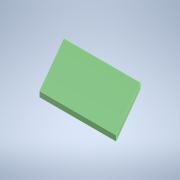
# Autodesk Inventor part: FactionSpecial_Council_Homel
Saved by Autodesk Inventor 2021 (Build 250183000, 183)
## iProperties
Created: 2023-03-16
Part Number: FactionSpecial_Council_Homel
Material: ABS Plastic
Document SubType Name: Modeling
Designer: Bradley
Density: 1.06 g/cm^3
Appearance: Smooth - Dark Forest Green
Author: Bradley
Autodesk Inventor part; units mm, degrees
ref_plane "YZ Plane" through (0, 0, 0) normal (1, 0, 0) x (0, 1, 0)
ref_plane "XZ Plane" through (0, 0, 0) normal (0, 1, 0) x (-1, 0, 0)
ref_plane "XY Plane" through (0, 0, 0) normal (0, 0, 1) x (1, 0, 0)
sketch "Sketch1" plane through (0, 0, 0) normal (0, 1, 0) x (-1, 0, 0)
  line L0 (-13.3945, -10.075) -> (13.3945, -10.075)
  line L1 (13.3945, -10.075) -> (1.7609, 10.075)
  line L2 (1.7609, 10.075) -> (-25.0281, 10.075)
  line L3 (-25.0281, 10.075) -> (-13.3945, -10.075)
  point P0 (0, 0)
  point P1 (0, -10.075)
  point P2 (7.5777, 0)
  dimension "d12" = 20.15
  dimension "d13" = 120
  dimension "d14" = 23.2
  constraints: 8 end point, 2 midpoint, 1 horizontal, 1 horizontal alignment, 1 parallel, 1 vertical alignment
  measures "d12" distance between parallel lines of L2 L0
  measures "d13" angle of L3 L0
  measures "d14" distance between parallel lines of L1 L3
extrude "Extrusion1" add sketch "Sketch1" along normal mid plane 1.9
body "Solid1"
